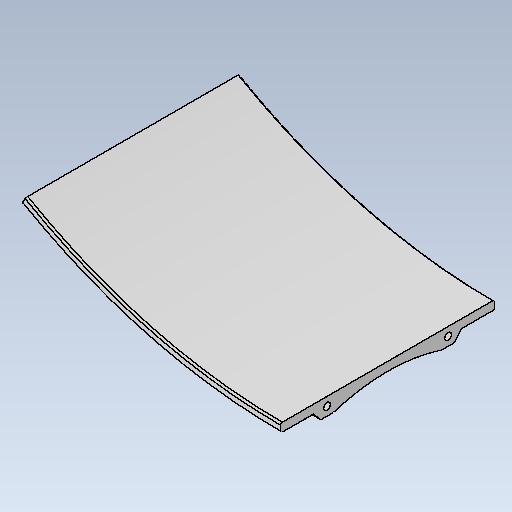
# Autodesk Inventor part: wheel_plate
Saved by Autodesk Inventor 2026.2 (Build 302298000, 298)
## iProperties
Created: 2026-01-18
Part Number: wheel_plate
Material: Generic
Document SubType Name: Modeling
Designer: gakut
Density: 1 g/cm^3
Appearance: Default
Author: gakut
## iProperties of the stored document wheel_plate_3DPrint.ipt
Created: 2026-01-26
Part Number: wheel_plate_3DPrint
Material: Generic
Document SubType Name: Modeling
Designer: gakut
Density: 1 g/cm^3
Appearance: Default
Author: gakut
Autodesk Inventor part; units mm, degrees
ref_plane "YZ Plane" through (0, 0, 0) normal (1, 0, 0) x (0, 1, 0)
ref_plane "XZ Plane" through (0, 0, 0) normal (0, 1, 0) x (-1, 0, 0)
ref_plane "XY Plane" through (0, 0, 0) normal (0, 0, 1) x (1, 0, 0)
sketch "Sketch2" plane through (0, 0, 0) normal (0, 0, 1) x (1, 0, 0)
  line L0 (-125, -5) -> (125, -5)
  line L1 (125, -5) -> (125, 5)
  line L2 (125, 5) -> (-125, 5)
  line L3 (-125, 5) -> (-125, -5)
  line L4 (-125, -5) -> (125, 5) construction
  line L5 (125, -5) -> (-125, 5) construction
  line L6 (-86.609004, -5) -> (-78.218007, -15)
  line L7 (78.218007, -15) -> (86.609004, -5)
  arc A0 (63.218007, -15) -> (-63.218007, -15) centre (0, -209.825823) ccw
  line L8 (-78.218007, -15) -> (-63.218007, -15)
  line L9 (63.218007, -15) -> (78.218007, -15)
  line L10 (101.609004, -5) -> (110, -15)
  line L11 (110, -15) -> (125, -15)
  line L12 (125, -15) -> (125, -5)
  line L13 (-101.609004, -5) -> (-110, -15)
  line L14 (-110, -15) -> (-125, -15)
  line L15 (-125, -15) -> (-125, -5)
  line L16 (125, 0) -> (-125, 0)
  line L17 (101.609004, 5) -> (110, 15)
  line L18 (110, 15) -> (125, 15)
  line L19 (125, 15) -> (125, 5)
  line L20 (-101.609004, 5) -> (-110, 15)
  line L21 (-110, 15) -> (-125, 15)
  line L22 (-125, 15) -> (-125, 5)
  point P0 (0, 0)
  dimension "d10" = 250
  dimension "d15" = 50
  dimension "d16" = 50
  dimension "d17" = 15
  dimension "d18" = 15
  dimension "d25" = 50
  dimension "d26" = 50
  dimension "d27" = 15
  dimension "d28" = 15
  dimension "d29" = 15
  dimension "d30" = 15
  dimension "d31" = 10
  dimension "d32" = 10
  constraints: 46 end point, 6 symmetric about line, 5 horizontal, 4 equal length, 4 midpoint, 4 point on line, 3 collinear, 2 point on circle, 1 centre point, 1 perpendicular, 1 tangent
  measures "d10" distance of L1.end L2.end
  measures "d15" angle of L0 L6
  measures "d16" angle of L0 L7
  measures "d17" distance of L8.end L6.end
  measures "d18" distance of L7.start L9.start
  measures "d25" angle of L10 L0
  measures "d26" angle of L13 L0
  measures "d27" distance of L10.end L11.end
  measures "d28" distance of L13.end L14.end
  measures "d29" distance of L6.start L13.start
  measures "d30" distance of L10.start L7.end
  measures "d31" distance between parallel lines of L0 L2
  measures "d32" distance between parallel lines of L14 L0
sketch "Sketch3" plane through (0, 0, 0) normal (1, 0, 0) x (0, 1, 0)
  arc A0 (80.384758, 300) -> (0, 0) centre (600, 0) ccw
  line L0 (600, 0) -> (0, 0) construction
  line L1 (80.384758, 300) -> (600, 0) construction
  dimension "d20" = 600
  dimension "d21" = 30
  dimension "d22" = 310.58285
  constraints: 4 end point, 2 point on circle, 1 centre point, 1 horizontal
  measures "d20" distance of L0.end L0.start
  measures "d21" angle of L0 L1
  measures "d22" distance of L0.end L1.start
sweep "Sweep1" add profiles "Sketch2" path "Sketch3" contours L3 L16 L1 L0 | L3 L2 L1 L16 | L0 A0 L8 L6 | L0 L7 L9 A0
sketch "Sketch4" plane through (125, 5, 0) normal (0, 0, -1) x (-1, 0, 0)
  line L0 (250, 0) -> (250, -10)
  line L1 (203.218007, -20) -> (188.218007, -20)
  line L2 (61.781993, -20) -> (46.781993, -20)
  point P0 (125, -5)
  point P1 (54.281993, -10)
  point P2 (195.718007, -10)
  point P3 (250, -5)
  point P4 (195.718007, -20)
  point P5 (54.281993, -20)
  point P6 (211.609004, -10)
  constraints: 3 midpoint, 2 horizontal alignment, 2 vertical alignment
hole "Hole1" at (-70.718007, -5, 0) at (70.718007, -5, 0) direction (0, 0, 1) diameter 8 depth 16
sketch "Sketch5" plane through (-125, 84.714885, 297.5) normal (0, 0.5, 0.8660254) x (1, 0, 0)
  line L0 (188.218007, -20) -> (203.218007, -20)
  line L1 (46.781993, -20) -> (61.781993, -20)
  point P0 (125, 75.384758)
  point P1 (54.281993, -10)
  point P2 (195.718007, -10)
  point P3 (250, -10)
  point P4 (195.718007, -20)
  point P5 (54.281993, -20)
  point P6 (211.609004, -10)
  constraints: 2 horizontal alignment, 2 midpoint, 2 vertical alignment
hole "Hole2" at (-70.718007, 76.054631, 302.5) at (70.718007, 76.054631, 302.5) direction (0, -0.5, -0.8660254) diameter 8 depth 16
fillet "Fillet1" radius 2 6 edges at (-125, 15.6149, 156.5855) (-125, 25.2741, 153.9973) (125, 25.2741, 153.9973) (125, 15.6149, 156.5855) (-78.218, 5.9556, 159.1737) (78.218, 5.9556, 159.1737)
equation "\"d15\" = d26"
equation "\"d16\" = d26"
equation "\"d17\" = d28"
equation "\"d18\" = d17"
equation "\"d25\" = d26"
equation "\"d27\" = d28"
equation "\"d30\" = d29"
body "Solid2"
